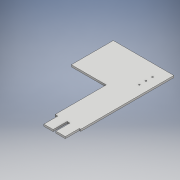
# Autodesk Inventor part: Arm
Saved by Autodesk Inventor 2018 (Build 220112000, 112)
## iProperties
Created: 2018-04-26
Part Number: Arm
Material: Generic
Document SubType Name: Modeling
Designer: HP
Density: 1 g/cm^3
Appearance: Default
Author: HP
Autodesk Inventor part; units mm, degrees
ref_plane "YZ Plane" through (0, 0, 0) normal (1, 0, 0) x (0, 1, 0)
ref_plane "XZ Plane" through (0, 0, 0) normal (0, 1, 0) x (-1, 0, 0)
ref_plane "XY Plane" through (0, 0, 0) normal (0, 0, 1) x (1, 0, 0)
sketch "Sketch4" plane through (0, 0, 0) normal (0, 0, 1) x (1, 0, 0)
  line L0 (0, 0) -> (65, 0)
  line L1 (65, 0) -> (65, 100)
  line L2 (65, 100) -> (0, 100)
  line L3 (0, 100) -> (0, 0)
  line L4 (1.5, 0) -> (11.5, 0)
  line L5 (11.5, 0) -> (11.5, -15)
  line L6 (11.5, -15) -> (1.5, -15)
  line L7 (1.5, -15) -> (1.5, 0)
  line L8 (14.5, 0) -> (24.5, 0)
  line L9 (24.5, 0) -> (24.5, -15)
  line L10 (24.5, -15) -> (14.5, -15)
  line L11 (14.5, -15) -> (14.5, 0)
  line L12 (32.5, 0) -> (42.5, 0)
  line L13 (27.5, 0) -> (37.5, 0)
  line L14 (37.5, 0) -> (37.5, -15)
  line L15 (37.5, -15) -> (27.5, -15)
  line L16 (27.5, -15) -> (27.5, 0)
  line L17 (40.5, 0) -> (50.5, 0)
  line L18 (50.5, 0) -> (50.5, -15)
  line L19 (50.5, -15) -> (40.5, -15)
  line L20 (40.5, -15) -> (40.5, 0)
  line L21 (53.5, 0) -> (63.5, 0)
  line L22 (63.5, 0) -> (63.5, -15)
  line L23 (63.5, -15) -> (53.5, -15)
  line L24 (53.5, -15) -> (53.5, 0)
  dimension "d39" = 65
  dimension "d40" = 100
  dimension "d41" = 10
  dimension "d42" = 15
  dimension "d43" = 1.5
  dimension "d44" = 10
  dimension "d45" = 15
  dimension "d47" = 3
  dimension "d49" = 10
  dimension "d50" = 10
  dimension "d51" = 15
  dimension "d52" = 3
  dimension "d53" = 3
  dimension "d54" = 10
  dimension "d55" = 15
  dimension "d56" = 3
  constraints: 50 end point, 12 parallel, 7 horizontal, 6 perpendicular, 5 point on line, 1 midpoint
  measures "d39" distance of L2.end L1.end
  measures "d40" distance of L1.end L0.end
  measures "d41" distance of L5.end L6.end
  measures "d42" distance of L4.end L5.end
  measures "d43" distance between parallel lines of L3 L7
  measures "d44" distance of L9.end L10.end
  measures "d45" distance of L8.end L9.end
  measures "d47" distance between parallel lines of L5 L11
  measures "d49" distance of L14.end L15.end
  measures "d50" distance of L18.end L19.end
  measures "d51" distance of L17.end L18.end
  measures "d52" distance between parallel lines of L9 L16
  measures "d53" distance between parallel lines of L20 L14
  measures "d54" distance of L22.end L23.end
  measures "d55" distance of L21.end L22.end
  measures "d56" distance between parallel lines of L18 L24
extrude "Extrusion4" add sketch "Sketch4" along normal blind 2
sketch "Sketch5" plane through (0, 0, 2) normal (0, 0, 1) x (1, 0, 0)
  circle A0 centre (55, 80) radius 0.75
  line L0 (65, 100) -> (0, 100) projected
  line L1 (65, 0) -> (65, 100) projected
  circle A1 centre (55, 72.9) radius 0.75
  circle A2 centre (55, 87.1) radius 0.75
  point P0 (0, 0)
  dimension "d59" = 1.5
  dimension "d60" = 20
  dimension "d61" = 10
  dimension "d62" = 1.5
  dimension "d63" = 7.1
  dimension "d64" = 1.5
  dimension "d65" = 7.1
  constraints: 3 centre point
  measures "d59" diameter of A0
  measures "d60" distance from line of L0 A0.centre
  measures "d61" distance from line of L1 A0.centre
  measures "d62" diameter of A1
  measures "d63" distance of A1.centre A0.centre
  measures "d64" diameter of A2
  measures "d65" distance of A0.centre A2.centre
extrude "Extrusion5" cut sketch "Sketch5" against normal blind 2
sketch "Sketch6" plane through (0, 0, 2) normal (0, 0, 1) x (1, 0, 0)
  line L0 (0, -15) -> (37.5, -15)
  line L1 (37.5, -15) -> (37.5, 55)
  line L2 (37.5, 55) -> (0, 55)
  line L3 (0, 55) -> (0, -15)
  point P0 (0, 0)
  dimension "d68" = 37.5
  dimension "d69" = 70
  constraints: 8 end point, 2 parallel, 1 horizontal, 1 perpendicular
  measures "d68" distance of L2.end L1.end
  measures "d69" distance of L1.end L0.end
extrude "Extrusion6" cut sketch "Sketch6" against normal blind 2
body "Solid2"
